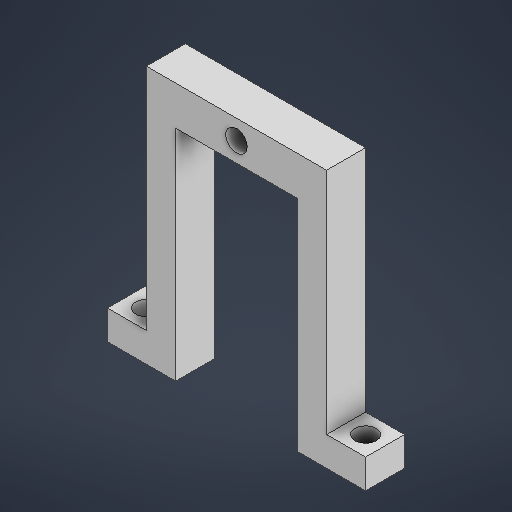
# Autodesk Inventor part: mocowanie-serwomechanizmy
Saved by Autodesk Inventor 2026.2 (Build 302298010, 298A)
## iProperties
Created: 2026-04-19
Part Number: mocowanie-serwomechanizmy
Material: Ogólny
Document SubType Name: Modeling
Designer: macie
Density: 1 g/cm^3
Appearance: Domyślna
Author: macie
Autodesk Inventor part; units mm, degrees
ref_plane "YZ Plane" through (0, 0, 0) normal (1, 0, 0) x (0, 1, 0)
ref_plane "XZ Plane" through (0, 0, 0) normal (0, 1, 0) x (-1, 0, 0)
ref_plane "XY Plane" through (0, 0, 0) normal (0, 0, 1) x (1, 0, 0)
sketch "Szkic1" plane through (0, 0, 0) normal (0, 1, 0) x (-1, 0, 0)
  line L0 (1.5, 2) -> (-1.5, 2)
  line L1 (-1.5, 2) -> (-1.5, -2)
  line L2 (-1.5, -2) -> (1.5, -2)
  line L3 (1.5, -2) -> (1.5, 2)
  line L4 (1.5, 2) -> (-1.5, -2) construction
  line L5 (-1.5, 2) -> (1.5, -2) construction
  point P0 (0, 0)
  dimension "d0" = 4
  dimension "d1" = 3
  constraints: 12 end point, 2 midpoint, 2 parallel, 1 horizontal, 1 perpendicular
  measures "d0" distance between parallel lines of L2 L0
  measures "d1" distance between parallel lines of L1 L3
extrude "Wyciągnięcie proste1" add sketch "Szkic1" along normal blind 26.5
sketch "Szkic2" plane through (-1.5, 0, -2) normal (-1, 0, 0) x (0, 0, 1)
  line L0 (4, 26.5) -> (0, 26.5) projected
  line L1 (4, 0) -> (4, 26.5) projected
  line L2 (0, 26.5) -> (4, 26.5)
  line L3 (4, 26.5) -> (4, 22.5)
  line L4 (4, 22.5) -> (0, 22.5)
  line L5 (0, 22.5) -> (0, 26.5)
  point P0 (2, 0)
  dimension "d4" = 4
  constraints: 8 end point, 2 parallel, 1 horizontal, 1 perpendicular, 1 point on line
  measures "d4" distance between parallel lines of L4 L0
extrude "Wyciągnięcie proste2" add sketch "Szkic2" along normal blind 15.5
sketch "Szkic3" plane through (-1.5, 22.5, -2) normal (0, -1, 0) x (1, 0, 0)
  line L0 (3, 4) -> (-15.5, 4) projected
  line L1 (3, 0) -> (-15.5, 0) projected
  line L2 (-15.5, 4) -> (-12.5, 4)
  line L3 (-12.5, 4) -> (-12.5, 0)
  line L4 (-12.5, 0) -> (-15.5, 0)
  line L5 (-15.5, 0) -> (-15.5, 4)
  point P0 (1.5, 2)
  dimension "d7" = 3
  constraints: 8 end point, 2 parallel, 1 horizontal, 1 perpendicular, 1 point on line
  measures "d7" distance between parallel lines of L3 L5
extrude "Wyciągnięcie proste3" add sketch "Szkic3" along normal blind 22.5
sketch "Szkic4" plane through (1.5, 0, 2) normal (1, 0, 0) x (0, 0, -1)
  line L0 (4, 0) -> (0, 0) projected
  line L1 (4, 22.5) -> (4, 0) projected
  line L2 (0, 0) -> (4, 0)
  line L3 (4, 0) -> (4, 3)
  line L4 (4, 3) -> (0, 3)
  line L5 (0, 3) -> (0, 0)
  point P0 (2, 0)
  dimension "d10" = 3
  constraints: 8 end point, 2 parallel, 1 horizontal, 1 perpendicular, 1 point on line
  measures "d10" distance between parallel lines of L0 L4
extrude "Wyciągnięcie proste4" add sketch "Szkic4" along normal blind 4
sketch "Szkic5" plane through (-17, 0, -2) normal (-1, 0, 0) x (0, 0, 1)
  line L0 (0, 0) -> (4, 0) projected
  line L1 (4, 3) -> (0, 3) projected
  line L2 (0, 0) -> (4, 0)
  line L3 (4, 0) -> (4, 3)
  line L4 (4, 3) -> (0, 3)
  line L5 (0, 3) -> (0, 0)
  point P0 (2, 0)
  constraints: 8 end point, 2 parallel, 1 horizontal, 1 perpendicular
extrude "Wyciągnięcie proste5" add sketch "Szkic5" along normal blind 4
sketch "Szkic6" plane through (1.5, 3, 2) normal (0, 1, 0) x (1, 0, 0)
  line L0 (0, 0) -> (4, 0) projected
  line L1 (0, 4) -> (4, 4) projected
  line L2 (4, 0) -> (0, 4)
  line L3 (4, 0) -> (4, 4) projected
  line L4 (0, 0) -> (4, 4)
  circle A0 centre (2, 2) radius 1.1
  line L5 (-22.5, 4) -> (-22.5, 0) projected
  line L6 (-18.5, 4) -> (-18.5, 0) projected
  line L7 (-22.5, 0) -> (-18.5, 4)
  line L8 (-18.5, 4) -> (-22.5, 4) projected
  line L9 (-18.5, 0) -> (-22.5, 4)
  circle A1 centre (-20.5, 2) radius 1.1
  point P0 (-1.5, 2)
  dimension "d15" = 2.2
  dimension "d16" = 2.2
  constraints: 8 end point, 2 centre point, 2 midpoint
  measures "d15" diameter of A0
  measures "d16" diameter of A1
hole "Otwór1" at (3.5, 3, 0) at (-19, 3, 0) direction (0, -1, 0) diameter 2.2 end through all
sketch "Szkic7" plane through (1.5, 26.5, -2) normal (0, 0, -1) x (-1, 0, 0)
  line L0 (3, -4) -> (15.5, -4) projected
  line L1 (3, -4) -> (3, 0)
  line L2 (0, 0) -> (18.5, 0) projected
  line L3 (15.5, -4) -> (15.5, -26.5) projected
  line L4 (3, 0) -> (15.5, -4)
  line L5 (15.5, -4) -> (15.5, 0)
  line L6 (15.5, 0) -> (3, -4)
  point P0 (1.5, -26.5)
  point P1 (9.25, -2)
  constraints: 8 end point, 2 point on line, 1 midpoint, 1 perpendicular, 1 vertical
hole "Otwór3" at (-7.75, 24.5, -2) direction (0, 0, 1) diameter 2.2 end through all
